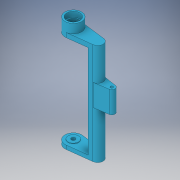
# Autodesk Inventor part: Servo-Arm-Lip
Saved by Autodesk Inventor 2018.3 (Build 223284000, 284)
## iProperties
Created: 2018-02-17
Part Number: Servo-Arm-Lip
Material: Generisch
Document SubType Name: Modeling
Designer: JochenAlt
Density: 1 g/cm^3
Appearance: Vorgabe
Author: JochenAlt
Autodesk Inventor part; units mm, degrees
ref_plane "YZ Plane" through (0, 0, 0) normal (1, 0, 0) x (0, 1, 0)
ref_plane "XZ Plane" through (0, 0, 0) normal (0, 1, 0) x (-1, 0, 0)
sketch "Skizze1" plane through (0, 0, 0) normal (0, 0, 1) x (1, 0, 0)
  line L0 (0, 5.6) -> (0, -5.6) construction
  line L1 (-9.12, 0) -> (26.72, 0) construction
  circle A0 centre (0, 0) radius 2
  circle A1 centre (9.5, 0) radius 1
  circle A2 centre (16, 0) radius 1
  circle A3 centre (19, 0) radius 1
  arc A4 (19.191579, -2.592932) -> (19.191579, 2.592932) centre (19, 0) ccw
  arc A5 (0.294737, 3.989126) -> (0.294737, -3.989126) centre (0, 0) ccw
  line L2 (0.294737, 3.989126) -> (19.191579, 2.592932)
  line L3 (0.294737, -3.989126) -> (19.191579, -2.592932)
  circle A6 centre (12.8, 0) radius 1
  circle A7 centre (0, 0) radius 4
  point P0 (0.526316, 3.965223)
  point P1 (0.657895, -1.888697)
  point P2 (0.657895, 1.888697)
  dimension "d0" = 9.5
  dimension "d1" = 16
  dimension "d2" = 19
  dimension "d3" = 5.2
  dimension "d4" = 2
  dimension "d5" = 4
  dimension "d6" = 8
  dimension "d17" = 12.8
  constraints: 7 centre point, 7 point on circle, 4 coincident, 4 end point, 4 point on line, 4 tangent, 3 equal radius, 3 other
  measures "d0" distance of A1.centre point (0, 0)
  measures "d1" distance of point (0, 0) A2.centre
  measures "d2" distance of A3.centre point (0, 0)
  measures "d3" diameter of A4
  measures "d4" diameter of A3
  measures "d5" diameter of A0
  measures "d6" diameter of A5
  measures "d17" distance of A6.centre point (0, 0)
extrude "Extrusion1" add sketch "Skizze1" along normal blind 1.8
extrude "Extrusion2" add sketch "Skizze1" against normal blind 2.7 contours A5 A7
sketch "Skizze6" plane through (0, 0, 0) normal (0, 0, 1) x (1, 0, 0)
  line L0 (0.294737, 3.989126) -> (19.191579, 2.592932) construction
  arc A0 (19.191579, -2.592932) -> (19.191579, 2.592932) centre (19, 0) ccw construction
  line L1 (19.191579, -2.592932) -> (0.294737, -3.989126) construction
  arc A1 (0.294737, -3.989126) -> (0.294737, 3.989126) centre (0, 0) ccw construction
  circle A2 centre (12.8, 0) radius 1 construction
  circle A3 centre (19, 0) radius 1 construction
  circle A4 centre (16, 0) radius 1 construction
  circle A5 centre (9.5, 0) radius 1 construction
  arc A6 (19.198947, -2.69266) -> (19.198947, 2.69266) centre (19, 0) ccw
  line L2 (19.198947, 2.69266) -> (0.302105, 4.088855)
  circle A7 centre (9.5, 0) radius 1 construction
  circle A8 centre (19, 0) radius 1
  line L3 (-14.3, 0) -> (40.3, 0) construction
  line L4 (0.302104, -4.088855) -> (19.198947, -2.69266)
  circle A9 centre (0, 0) radius 2 construction
  circle A10 centre (0, 0) radius 1.25
  arc A11 (0.786842, 6.4522) -> (0.786842, -6.4522) centre (0, 0) ccw
  line L5 (19, 0) -> (30, 0) construction
  circle A12 centre (30, 0) radius 1.05
  circle A13 centre (30, 0) radius 2.5
  arc A14 (15.990551, -2.929713) -> (15.990551, 2.929713) centre (19, 0) ccw
  line L6 (19.649091, -4.14954) -> (30.386364, -2.469964)
  line L7 (19.649091, 4.14954) -> (30.386364, 2.469964)
  line L8 (0.786842, -6.4522) -> (19.508421, -4.169114)
  arc A15 (15.990551, 2.929713) -> (15.990551, -2.929713) centre (19, 0) ccw
  line L9 (15.990551, -2.929713) -> (16.191031, -4.573667)
  line L10 (19.508421, 4.169114) -> (0.786842, 6.4522)
  line L11 (16.191031, 4.573667) -> (15.990551, 2.929713)
  line L12 (30, 0) -> (0, 0) construction
  arc A16 (0.302105, 4.088855) -> (0.302104, -4.088855) centre (0, 0) ccw
  arc A17 (0.302104, -4.088855) -> (0.302105, 4.088855) centre (0, 0) ccw
  circle A18 centre (0, 0) radius 1.5
  dimension "d106" = 2.5
  dimension "d116" = 0.1
  dimension "d235" = 6.5
  dimension "d250" = 2.1
  dimension "d251" = 5
  dimension "d252" = 180
  dimension "d253" = 1.5
  dimension "d261" = 30
  dimension "d262" = 3
  constraints: 20 end point, 18 point on circle, 13 centre point, 11 tangent, 9 coincident, 4 point on line, 2 concentric, 2 perpendicular, 1 parallel
  measures "d106" diameter of A10
  measures "d116" distance between parallel lines of L4 L1
  measures "d235" radius of A11
  measures "d250" diameter of A12
  measures "d251" diameter of A13
  measures "d252" angle of L3 L5
  measures "d253" radial gap between concentric circles of A14 A6
  measures "d261" distance of L12.end L12.start
  measures "d262" diameter of A18
extrude "Extrusion11" add sketch "Skizze6" along normal blind 2 separate body contours A6 L2 A14 L4 | L9 L8 A11 L10 L11 L2 A16 L4 | A14 L8 L9 | L11 L10 A14
extrude "Extrusion12" add sketch "Skizze6" along normal blind 1.5 from surface at 2 contours L4 A15 L2 A6 | A6 L2 A14 L4 | L9 L8 A11 L10 L11 L2 A16 L4 | L4 A17 L2 A15 | A14 L8 L9 | L11 L10 A14 | A16 A17 | A8 | A18
sketch "Skizze18" plane through (0, 0, 3.5) normal (0, 0, 1) x (0.9999808, 0.0061906, 0)
  circle A0 centre (0, 0) radius 5.15
  circle A1 centre (0, 0) radius 6.5
  circle A2 centre (0, 0) radius 4
  line L0 (19.482238, -4.289803) -> (0.746884, -6.456947) construction
  arc A3 (19.482238, -4.289803) -> (19.533857, 4.048264) centre (18.999636, -0.117622) ccw construction
  line L1 (0.82677, 6.447205) -> (19.533857, 4.048264) construction
  arc A4 (0.82677, 6.447205) -> (0.746884, -6.456947) centre (0, 0) ccw construction
  point P0 (-6.499875, 0.040239)
  dimension "d183" = 10.3
  dimension "d192" = 8
  constraints: 3 coincident, 2 centre point, 1 point on circle, 3 other
  measures "d183" diameter of A0
  measures "d192" diameter of A2
extrude "Extrusion29" add sketch "Skizze18" along normal blind 3 contours A0 | A1
extrude "Extrusion28" add sketch "Skizze18" along normal blind 4 from surface at 3 contours A1
extrude "Extrusion37" add sketch "Skizze6" against normal blind 72.5 contours A6 L2 A14 L4 | A14 L8 L9 | L11 L10 A14
extrude "Extrusion34" add sketch "Skizze6" against normal blind 3 from surface at -72.5 contours L4 A15 L2 A6 | A6 L2 A14 L4 | L9 L8 A11 L10 L11 L2 A16 L4 | L4 A17 L2 A15 | A14 L8 L9 | L11 L10 A14 | A16 A17 | A8
extrude "Extrusion35" add sketch "Skizze6" along normal blind 0.5 from surface at -72.5 contours A16 A17
ref_plane "Arbeitsebene10" through (0, 0, -30.5) normal (0, 0, 1) x (1, 0, 0)
extrude "Extrusion36" add sketch "Skizze6" along normal mid plane 17 from surface at -30.5 contours A14 L7 A13 L6 | A13
sketch "Skizze23" plane through (17.436389, -3.898092, -30.5) normal (0, 0, 1) x (0.9281172, -0.3722882, 0)
  line L0 (-1.702423, 0.360501) -> (-0.90433, -1.090646)
  line L1 (-14.501866, -8.568942) -> (-0.90433, -1.090646)
  arc A0 (-19.306022, 3.407852) -> (-14.501866, -8.568942) centre (-17.634226, -2.873477) ccw
  line L2 (-4.309775, 7.399153) -> (-19.306022, 3.407852)
  line L3 (-4.309775, 7.399153) -> (-3.883819, 5.798734)
  line L4 (-18.876069, 1.03393) -> (-3.883819, 5.798734)
  line L5 (-1.702423, 0.360501) -> (-15.831605, -6.555943)
  line L6 (-0.817799, 6.77317) -> (-3.883819, 5.798734)
  arc A1 (1.187092, 1.774961) -> (-0.817799, 6.77317) centre (0, 4.2) ccw
  line L7 (0.21672, 6.891288) -> (0.440086, 9.37592)
  arc A2 (-18.876069, 1.03393) -> (-15.831605, -6.555943) centre (-17.634226, -2.873477) ccw
  line L8 (-4.309775, 7.399153) -> (-3.883819, 5.798734)
  line L9 (-4.309775, 7.399153) -> (-4.486884, 8.064591)
  line L10 (-4.486884, 8.064591) -> (0.440086, 9.37592)
  constraints: 6 end point, 2 collinear, 1 perpendicular, 1 point on circle
extrude "Extrusion40" cut sketch "Skizze23" along normal mid plane 7
fillet "Rundung10" radius 3 2 edges at (20.5913, 3.1793, -27) (20.5913, 3.1793, -34)
chamfer "Fase8" distance 1 distance2 1.5 11 edges at (20.9795, 3.9414, -30.5) (20.627, 3.9966, -28.6144) (19.5797, 4.1598, -27.4968) (19.5083, 4.1691, -27.4533) (18.7041, 4.2672, -27.1155) (17.0119, 4.4736, -27) (20.627, 3.9966, -32.3856) (19.5083, 4.1691, -33.5467) (19.5797, 4.1598, -33.5032) (18.7041, 4.2672, -33.8845) (17.0119, 4.4736, -34) measured on face at (19.5954, 4.1576, -33.5286) measured on face at (18.8328, 4.2515, -26.6327) measured on face at (17.0119, 4.4736, -34.5) measured on face at (21.0602, 3.9288, -28.3741) measured on face at (19.4016, 3.6875, -27.5345) measured on face at (18.8328, 4.2515, -34.3673) measured on face at (21.4735, 3.8642, -30.5) measured on face at (17.0119, 4.4736, -26.5) measured on face at (21.0602, 3.9288, -32.6259) measured on face at (19.4016, 3.6875, -33.4655) measured on face at (19.5954, 4.1576, -27.4714)
